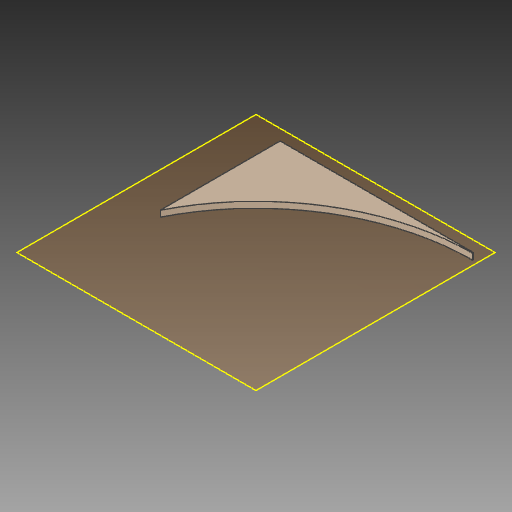
# Autodesk Inventor part: Cyclone Inlet
Saved by Autodesk Inventor 2018.2 (Build 222227000, 227)
## iProperties
Created: 2018-02-08
Part Number: Cyclone Inlet
Material: Generic
Document SubType Name: Modeling
Designer: Rus
Density: 1 g/cm^3
Appearance: Default
Author: Rus
Autodesk Inventor part; units mm, degrees
ref_plane "YZ Plane" through (0, 0, 0) normal (1, 0, 0) x (0, 1, 0)
ref_plane "XZ Plane" through (0, 0, 0) normal (0, 1, 0) x (-1, 0, 0)
ref_plane "XY Plane" through (0, 0, 0) normal (0, 0, 1) x (1, 0, 0)
ref_plane "Work Plane1" through (-228.0882, -76.2, -228.6) normal (0, 1, 0) x (-1, 0, 0)
sketch "Sketch2" plane through (-228.0882, -76.2, -228.6) normal (0, 1, 0) x (-1, 0, 0)
  circle A0 centre (-228.6, 228.6) radius 227.5764 construction
  circle A1 centre (-228.6, 228.6) radius 228.6 construction
  arc A2 (-228.6, 1.0236) -> (-25.4, 126.1267) centre (-228.6, 228.6) ccw construction
  arc A3 (-228.6, 0) -> (-25.4, 123.8731) centre (-228.6, 228.6) ccw construction
  line L0 (-228.6, 0) -> (-25.4, 0)
  arc A4 (-228.6, 1.0236) -> (-25.4, 126.1267) centre (-228.6, 228.6) ccw
  line L1 (-228.6, 228.6) -> (-25.4, 126.1267) construction
  line L2 (-228.6, 228.6) -> (-228.6, 1.0236) construction
  line L3 (-25.4, 126.1267) -> (-25.4, 0)
  line L4 (-228.6, 0) -> (-228.6, 1.0236)
  line L5 (-228.6, 0) -> (-228.6, 1.0236) projected
  line L6 (-25.4, 123.8731) -> (-25.4, 126.1267) projected
  point P0 (-228.0882, 228.6)
  point P1 (-1.0236, 228.6)
  point P2 (0, 228.6)
  point P3 (-228.6, 228.6)
  point P4 (-228.6, 228.6)
  dimension "d14" = 203.2
  constraints: 10 end point, 3 point on circle, 2 tangent, 1 centre point, 1 horizontal, 1 vertical
  measures "d14" distance of L0.start L0.end
extrude "Extrusion1" add sketch "Sketch2" against normal blind 6.35
body "Solid2"
